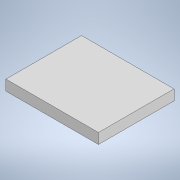
# Autodesk Inventor part: rx5808
Saved by Autodesk Inventor 2020 (Build 240168000, 168)
## iProperties
Created: 2020-03-15
Part Number: rx5808
Material: Generic
Document SubType Name: Modeling
Designer: erwin
Density: 1 g/cm^3
Appearance: Default
Author: erwin
Autodesk Inventor part; units mm, degrees
ref_plane "YZ Plane" through (0, 0, 0) normal (1, 0, 0) x (0, 1, 0)
ref_plane "XZ Plane" through (0, 0, 0) normal (0, 1, 0) x (-1, 0, 0)
ref_plane "XY Plane" through (0, 0, 0) normal (0, 0, 1) x (1, 0, 0)
sketch "Sketch1" plane through (0, 0, 0) normal (0, 1, 0) x (-1, 0, 0)
  line L0 (-14.2, -11.6) -> (14.2, -11.6)
  line L1 (14.2, -11.6) -> (14.2, 11.6)
  line L2 (14.2, 11.6) -> (-14.2, 11.6)
  line L3 (-14.2, 11.6) -> (-14.2, -11.6)
  line L4 (-14.2, -11.6) -> (14.2, 11.6) construction
  line L5 (14.2, -11.6) -> (-14.2, 11.6) construction
  point P0 (0, 0)
  dimension "d0" = 28.4
  dimension "d1" = 23.2
  constraints: 12 end point, 2 midpoint, 2 parallel, 1 horizontal, 1 perpendicular
  measures "d0" distance of L2.end L1.end
  measures "d1" distance of L1.end L0.end
extrude "Extrusion1" add sketch "Sketch1" along normal blind 3.2
body "Solid1"
